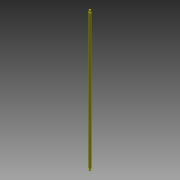
# Autodesk Inventor part: 载板连接销
Saved by Autodesk Inventor 2015 (Build 190159000, 159)
## iProperties
Created: 2017-05-02
Part Number: 载板连接销
Material: 常规
Document SubType Name: Modeling
Designer: Administrator
Density: 1 g/cm^3
Appearance: 黄色
Author: Administrator
Autodesk Inventor part; units mm, degrees
ref_plane "YZ Plane" through (0, 0, 0) normal (1, 0, 0) x (0, 1, 0)
ref_plane "XZ Plane" through (0, 0, 0) normal (0, 1, 0) x (-1, 0, 0)
ref_plane "XY Plane" through (0, 0, 0) normal (0, 0, 1) x (1, 0, 0)
sketch "草图1" plane through (0, 0, 0) normal (0, 0, 1) x (1, 0, 0)
  circle A0 centre (0, 0) radius 5
  dimension "d0" = 10
  constraints: 1 centre point, 1 coincident
  measures "d0" diameter of A0
extrude "拉伸1" add sketch "草图1" along normal mid plane 530
sketch "草图2" plane through (0, 0, 0) normal (0, 1, 0) x (-1, 0, 0)
  arc A0 (4.5149, 268.9403) -> (5, 265) centre (5, 267) ccw
  line L0 (5, 265) -> (-5, 265) projected
  line L1 (3, 275) -> (4.5149, 268.9403)
  line L2 (3, 275) -> (0, 275)
  line L3 (0, 275) -> (0, 265)
  line L4 (5, 265) -> (0, 265)
  point P0 (0, 0)
  dimension "d4" = 2
  dimension "d5" = 2
  dimension "d7" = 10
  dimension "d10" = 5
  dimension "d11" = 3
  constraints: 8 end point, 3 point on line, 2 point on circle, 1 centre point, 1 collinear, 1 horizontal, 1 midpoint
  measures "d4" distance from line of L0 A0.centre
  measures "d5" radius of A0
  measures "d7" distance of L2.end L3.end
  measures "d10" distance from line of L3 A0.centre
  measures "d11" distance of L1.start L2.end
revolve "旋转1" add sketch "草图2" angle 360 about axis through (0, 0, 275) along (0, 0, -1)
mirror "镜像1" about plane through (0, 0, 0) normal (0, 0, 1) of "旋转1"
